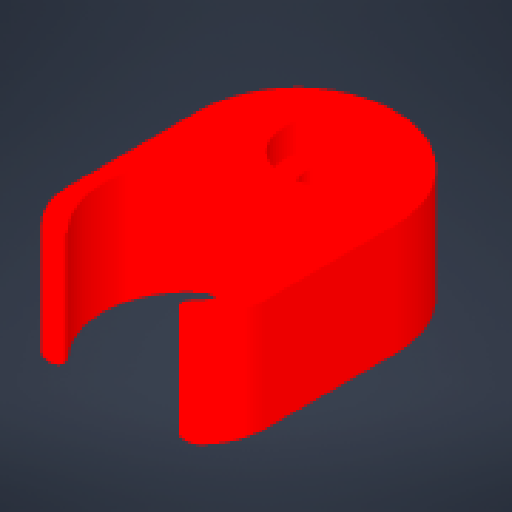
# Autodesk Inventor part: Z Stage Motor Clamp V5
Saved by Autodesk Inventor 2023.4 (Build 274418000, 418)
## iProperties
Created: 2024-05-29
Part Number: Z Stage Motor Clamp V5
Material: Generic
Document SubType Name: Modeling
Designer: xSibe
Density: 1 g/cm^3
Appearance: Plastic Red
Author: xSibe
Autodesk Inventor part; units mm, degrees
ref_plane "YZ Plane" through (0, 0, 0) normal (1, 0, 0) x (0, 1, 0)
ref_plane "XZ Plane" through (0, 0, 0) normal (0, 1, 0) x (-1, 0, 0)
sketch "Sketch1" plane through (0, 0, 0) normal (0, 1, 0) x (-1, 0, 0)
  line L0 (-113.9895, -20.65) -> (-113.9895, -0.1) projected
  line L1 (-105.9, -20.65) -> (-113.9895, -20.65) projected
  line L2 (-105.9, -20.65) -> (-105.9, -19.5) projected
  line L3 (-105.9, -19.5) -> (-112.525, -19.5) projected
  line L4 (-112.525, -19.5) -> (-112.525, 19.5) projected
  line L5 (-112.525, 19.5) -> (-73.775, 19.5) projected
  line L6 (-127.45, 19.9) -> (-115.3, 19.9) projected
  line L7 (-115.3, 19.9) -> (-115.3, 9.9) projected
  line L8 (-115.3, 9.9) -> (-127.45, 9.9) projected
  line L9 (-127.45, 9.9) -> (-127.45, 19.9) projected
  line L10 (-124.5373, 9.9) -> (-126.375, 9.9) projected
  arc A0 (-124.8248, 9.9909) -> (-124.5373, 9.9) centre (-124.5373, 10.4) ccw projected
  arc A1 (-127.375, 14.9) -> (-124.8248, 9.9909) centre (-121.375, 14.9) ccw projected
  line L11 (-127.375, 10.9) -> (-127.375, 14.9) projected
  arc A2 (-127.375, 10.9) -> (-126.375, 9.9) centre (-126.375, 10.9) ccw projected
  line L12 (-127.375, 14.9) -> (-127.375, 18.9) projected
  arc A3 (-124.8248, 19.8091) -> (-127.375, 14.9) centre (-121.375, 14.9) ccw projected
  arc A4 (-124.5373, 19.9) -> (-124.8248, 19.8091) centre (-124.5373, 19.4) ccw projected
  line L13 (-126.375, 19.9) -> (-124.5373, 19.9) projected
  arc A5 (-126.375, 19.9) -> (-127.375, 18.9) centre (-126.375, 18.9) ccw projected
  line L14 (-118.2127, 19.9) -> (-116.375, 19.9) projected
  arc A6 (-117.9252, 19.8091) -> (-118.2127, 19.9) centre (-118.2127, 19.4) ccw projected
  arc A7 (-115.375, 14.9) -> (-117.9252, 19.8091) centre (-121.375, 14.9) ccw projected
  line L15 (-115.375, 18.9) -> (-115.375, 14.9) projected
  arc A8 (-115.375, 18.9) -> (-116.375, 19.9) centre (-116.375, 18.9) ccw projected
  line L16 (-115.375, 14.9) -> (-115.375, 10.9) projected
  arc A9 (-117.9252, 9.9909) -> (-115.375, 14.9) centre (-121.375, 14.9) ccw projected
  arc A10 (-118.2127, 9.9) -> (-117.9252, 9.9909) centre (-118.2127, 10.4) ccw projected
  line L17 (-116.375, 9.9) -> (-118.2127, 9.9) projected
  arc A11 (-116.375, 9.9) -> (-115.375, 10.9) centre (-116.375, 10.9) ccw projected
  arc A12 (-118.2127, 9.9) -> (-117.9252, 9.9909) centre (-118.2127, 10.4) ccw projected
  arc A13 (-117.9252, 9.9909) -> (-117.9252, 19.8091) centre (-121.375, 14.9) ccw projected
  arc A14 (-117.9252, 19.8091) -> (-118.2127, 19.9) centre (-118.2127, 19.4) ccw projected
  line L18 (-118.2127, 19.9) -> (-124.5373, 19.9) projected
  arc A15 (-124.5373, 19.9) -> (-124.8248, 19.8091) centre (-124.5373, 19.4) ccw projected
  arc A16 (-124.8248, 19.8091) -> (-124.8248, 9.9909) centre (-121.375, 14.9) ccw projected
  arc A17 (-124.8248, 9.9909) -> (-124.5373, 9.9) centre (-124.5373, 10.4) ccw projected
  line L19 (-124.5373, 9.9) -> (-118.2127, 9.9) projected
  line L20 (-73.775, 19.5) -> (-73.775, 20.65) projected
  line L21 (-115.3, 19.9) -> (-115.3, 9.9)
  line L22 (-115.3, 9.9) -> (-114.3, 9.9)
  line L23 (-114.3, 9.9) -> (-114.3, 19.9)
  line L24 (-114.3, 19.9) -> (-115.3, 19.9)
  line L25 (-121.375, 14.9) -> (-121.375, 19.9)
  arc A18 (-114.3, 16.3047) -> (-115.6679, 19.6071) centre (-118.9703, 16.3047) ccw
  arc A19 (-116.375, 19.9) -> (-117.9252, 19.8091) centre (-116.375, 6.6367) ccw
  line L26 (-127.45, 19.9) -> (-127.45, 9.9)
  line L27 (-127.45, 9.9) -> (-128.45, 9.9)
  line L28 (-128.45, 9.9) -> (-128.45, 19.9)
  line L29 (-128.45, 19.9) -> (-127.45, 19.9)
  arc A20 (-127.0821, 19.6071) -> (-128.45, 16.3047) centre (-123.7797, 16.3047) ccw
  arc A21 (-124.8248, 19.8091) -> (-126.375, 19.9) centre (-126.375, 6.6367) ccw
  line L30 (-114.3, 9.9) -> (-128.45, 9.9)
  line L31 (-128.45, 9.9) -> (-128.45, -0.1)
  line L32 (-128.45, -0.1) -> (-114.3, -0.1)
  line L33 (-114.3, -0.1) -> (-114.3, 9.9)
  line L34 (-121.375, 9.9) -> (-121.375, -0.1)
  circle A22 centre (-121.375, 4.9) radius 1.5
  circle A23 centre (-121.375, 4.9) radius 3
  arc A24 (-121.375, -0.1) -> (-114.3, 6.975) centre (-121.375, 6.975) ccw
  arc A25 (-128.45, 6.975) -> (-121.375, -0.1) centre (-121.375, 6.975) ccw
  line L35 (-128.9145, -0.1) -> (-128.9145, 20.65) projected
  line L36 (-128.9145, -0.1) -> (-113.9895, -0.1) projected
  line L37 (-128.9145, 20.65) -> (-73.775, 20.65) projected
  circle A26 centre (-121.375, 4.9163) radius 1.4375 projected
  point P0 (0, 0)
  point P1 (-135.6645, 14.9)
  dimension "d18" = 1
  dimension "d20" = 3
  dimension "d21" = 6
  dimension "d22" = 10
  constraints: 28 end point, 13 point on circle, 8 centre point, 7 symmetric about line, 7 tangent, 5 point on line, 4 midpoint, 4 parallel, 3 perpendicular, 1 coincident, 1 collinear, 2 other
  measures "d18" distance of L22.end L7.end
  measures "d20" diameter of A22
  measures "d21" diameter of A23
  measures "d22" distance of L28.start L31.end
ref_plane "Work Plane1" through (127.45, 59.5, 9.9) normal (0, 1, 0) x (1, 0, 0)
extrude "Extrusion1" add sketch "Sketch1" along normal blind 6 from surface at 59.5 contours A25 L31 L27 L8 L34 A23 | L34 A23 L8 L22 L33 A24 | A23 L34 A22 | L34 A22 A23 | L22 L7 A18 L23 | L28 A20 L9 L27 | L8 A11 L16 L15 A8 A18 L7 | L9 A20 A5 L12 L11 A2 L8 | L8 A10 A9 L16 A11 | L8 A2 L11 A1 A0 | A8 L15 A7 A19 | A5 A21 A3 L12
fillet "Fillet1" radius 0.5 2 edges at (117.9252, 62.5, 19.8091) (124.8248, 62.5, 19.8091)
sketch "Sketch2" plane through (118.1857, 65.5, 20.6175) normal (0, 1, 0) x (1, 0, 0)
  arc A0 (-0.2604, 10.6266) -> (-1.1435, 1.567) centre (3.1893, 5.7175) ccw projected
  arc A1 (0.0271, 10.7175) -> (-0.2604, 10.6266) centre (0.0271, 10.2175) ccw projected
  line L0 (6.3516, 10.7175) -> (0.0271, 10.7175) projected
  arc A2 (6.6391, 10.6266) -> (6.3516, 10.7175) centre (6.3516, 10.2175) ccw projected
  arc A3 (7.5222, 1.567) -> (6.6391, 10.6266) centre (3.1893, 5.7175) ccw projected
  circle A4 centre (3.1893, 15.7175) radius 3
  arc A5 (10.2643, 13.6425) -> (-3.8857, 13.6425) centre (3.1893, 13.6425) ccw projected
  line L1 (-3.8857, 4.3128) -> (-3.8857, 13.6425) projected
  arc A6 (-3.8857, 4.3128) -> (-2.5178, 1.0104) centre (0.7846, 4.3128) ccw projected
  arc A7 (-2.5178, 1.0104) -> (-1.8107, 0.7175) centre (-1.8107, 1.7175) ccw projected
  arc A8 (-1.8107, 0.7175) -> (-1.4926, 0.7213) centre (-1.8107, 13.9808) ccw projected
  arc A9 (7.8713, 0.7213) -> (8.1893, 0.7175) centre (8.1893, 13.9808) ccw projected
  arc A10 (8.1893, 0.7175) -> (8.8964, 1.0104) centre (8.1893, 1.7175) ccw projected
  arc A11 (8.8964, 1.0104) -> (10.2643, 4.3128) centre (5.5941, 4.3128) ccw projected
  line L2 (10.2643, 13.6425) -> (10.2643, 4.3128) projected
  line L3 (3.1893, 10.7175) -> (3.1893, 20.7175)
  arc A12 (7.5222, 1.567) -> (7.8713, 0.7213) centre (7.8833, 1.2212) ccw projected
  arc A13 (-1.4926, 0.7213) -> (-1.1435, 1.567) centre (-1.5046, 1.2212) ccw projected
  point P0 (-118.1857, 20.6175)
  dimension "d10" = 6
  constraints: 2 end point, 2 midpoint, 1 centre point, 1 point on circle
  measures "d10" diameter of A4
extrude "Extrusion2" add sketch "Sketch2" along normal blind 2 contours A0 A13 A8 A7 A6 L1 A5 L3 A4 L0 A1 | L3 A4 A5 L2 A11 A10 A9 A12 A3 A2 L0
body "Solid1"
